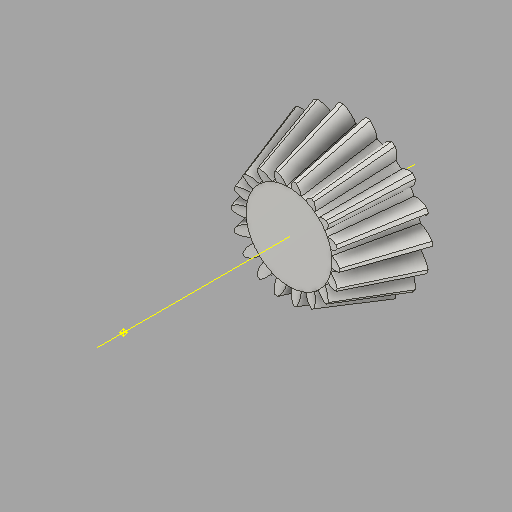
# Autodesk Inventor part: Bevel Gear1
Saved by Autodesk Inventor 2024 (Build 280153000, 153)
## iProperties
Created: 2024-04-12
Part Number: Bevel Gear1
Material: Steel, Mild
Document SubType Name: Modeling
Designer: Alex
Categories: <?xml version="1.0" encoding="UTF-16"?> <MemberInstance><Categories><FamilyTemplate><FamilyTemplateParameter ValueType="xs:double" Id="1" ObjectReferenceKey="da_z" ObjectType="kUserParameterObject"/><FamilyTemplateParameter ValueType="xs:double" Id="2" ObjectReferenceKey="da_b" ObjectType="kUserParameterObject"/><FamilyTemplateParameter ValueType="xs:double" Id="3" ObjectReferenceKey="da_beta" ObjectType="kUserParameterObject"/><FamilyTemplateParameter ValueType="xs:double" Id="4" ObjectReferenceKey="da_dae" ObjectType="kUserParameterObject"/><FamilyTemplateParameter ValueType="xs:double" Id="5" ObjectReferenceKey="da_ve" ObjectType="kUserParameterObject"/><FamilyTemplateParameter ValueType="xs:double" Id="6" ObjectReferenceKey="da_omega" ObjectType="kUserParameterObject"/><FamilyTemplateParameter ValueType="xs:string" Id="7" ObjectReferenceKey="EAIAABAAAAAAHwAAAAAAAIAAAAAAAAAA" ObjectType="83914240" SubObjectId="SurfaceGeometry"/></FamilyTemplate><ParamToTemplateMap><ParamToTemplate CategoryParameter="//CategoryParameter[@InternalName='046C89C9-8512-4d59-83FE-43B91F4F132A']" TemplateParameter="1"/><ParamToTemplate CategoryParameter="//CategoryParameter[@InternalName='2552DF32-E462-4b46-AEBF-C6C7768E72AC']" TemplateParameter="2"/><ParamToTemplate CategoryParameter="//CategoryParameter[@InternalName='C9EE641D-15FC-4fae-A226-E94C4372FDD7']" TemplateParameter="3"/><ParamToTemplate><ParamToTemplate CategoryParameter="//CategoryParameter[@InternalName='00B6519A-459B-49c7-AD84-2E56D39A5744']" ConstantValue="0.000000"/></ParamToTemplate><ParamToTemplate><ParamToTemplate CategoryParameter="//CategoryParameter[@InternalName='04B31F0E-C7A6-4894-AA32-9629BEFACF47']" ConstantValue="1.000000"/></ParamToTemplate><ParamToTemplate><ParamToTemplate CategoryParameter="//CategoryParameter[@InternalName='43CBEC2E-7847-49e7-A936-2F7889FCB2D9']" ConstantValue="0.200000"/></ParamToTemplate><ParamToTemplate><ParamToTemplate CategoryParameter="//CategoryParameter[@InternalName='B1EFC894-105D-4ebd-86BF-FA20ED196853']" ConstantValue="0.300000"/></ParamToTemplate><ParamToTemplate><ParamToTemplate CategoryParameter="//CategoryParameter[@InternalName='51175063-3D10-4879-93E8-6246FE8B403D']" ConstantValue="2060000000.000000"/></ParamToTemplate><ParamToTemplate><ParamToTemplate CategoryParameter="//CategoryParameter[@InternalName='A3A52E27-4454-46a9-B0BD-C932399B70AF']" ConstantValue="0.300000"/></ParamToTemplate><ParamToTemplate CategoryParameter="//CategoryParameter[@InternalName='2A200944-5A8C-41ca-B96E-8520D2E510F1']" TemplateParameter="4"/><ParamToTemplate><ParamToTemplate CategoryParameter="//CategoryParameter[@InternalName='1A637F62-92C8-44bc-B81F-10802510B579']" ConstantValue="2.794076"/></ParamToTemplate><ParamToTemplate CategoryParameter="//CategoryParameter[@InternalName='B52DD4BE-6863-48fb-BF58-89EF6F9EC65C']" TemplateParameter="5"/><ParamToTemplate><ParamToTemplate CategoryParameter="//CategoryParameter[@InternalName='3956BFF2-84D2-457d-93C2-9B0613DEBA67']" ConstantValue="4.168551"/></ParamToTemplate><ParamToTemplate CategoryParameter="//CategoryParameter[@InternalName='739CFA02-461B-4bf8-8049-181FCAD8B28F']" TemplateParameter="6"/><ParamToTemplate><ParamToTemplate CategoryParameter="//CategoryParameter[@InternalName='A27E999F-E2CE-4481-8A2A-EBF499C4C3C5']" ConstantValue="0.000000"/></ParamToTemplate><ParamToTemplate><ParamToTemplate CategoryParameter="//CategoryParameter[@InternalName='9E1B4470-B2D3-4ff1-B813-535BB4CDF51A']" ConstantValue="3520000.000000"/></ParamToTemplate><ParamToTemplate><ParamToTemplate CategoryParameter="//CategoryParameter[@InternalName='F8452263-BFF6-458c-9FB1-07C4B99E95CD']" ConstantValue="11400000.000000"/></ParamToTemplate><ParamToTemplate><ParamToTemplate CategoryParameter="//CategoryParameter[@InternalName='3E3BB259-FD49-497f-8171-6EBC954A3479']" ConstantValue="2.000000"/></ParamToTemplate><ParamToTemplate CategoryParameter="//CategoryParameter[@InternalName='27C3BAF2-7550-4e4b-AE2C-0DB134B7D9B7']" TemplateParameter="7"/></ParamToTemplateMap><Category DisplayName="Gear" InternalName="DC85795E-93AB-48d5-8EEE-5A27447B64BD" Mnemonic="Gear"><CategoryParameter DisplayName="z" InternalName="046C89C9-8512-4d59-83FE-43B91F4F132A" Mnemonic="z"/><CategoryParameter DisplayName="b" InternalName="2552DF32-E462-4b46-AEBF-C6C7768E72AC" Mnemonic="b"/><CategoryParameter DisplayName="||b|" InternalName="C9EE641D-15FC-4fae-A226-E94C4372FDD7" Mnemonic="beta"/><CategoryParameter DisplayName="x" InternalName="00B6519A-459B-49c7-AD84-2E56D39A5744" Mnemonic="x"/><CategoryParameter DisplayName="a*" InternalName="04B31F0E-C7A6-4894-AA32-9629BEFACF47" Mnemonic="a"/><CategoryParameter DisplayName="c*" InternalName="43CBEC2E-7847-49e7-A936-2F7889FCB2D9" Mnemonic="c"/><CategoryParameter DisplayName="r|.f|*" InternalName="B1EFC894-105D-4ebd-86BF-FA20ED196853" Mnemonic="rf"/><CategoryParameter DisplayName="E" InternalName="51175063-3D10-4879-93E8-6246FE8B403D" Mnemonic="E"/><CategoryParameter DisplayName="||m|" InternalName="A3A52E27-4454-46a9-B0BD-C932399B70AF" Mnemonic="mi"/><Category DisplayName="BevelGear" InternalName="0C98F69A-0C2B-4791-B2FE-7691BB227E77" Mnemonic="BevelGear"><CategoryParameter DisplayName="d|.ae|" InternalName="2A200944-5A8C-41ca-B96E-8520D2E510F1" Mnemonic="dae"/><CategoryParameter DisplayName="d|.ai|" InternalName="1A637F62-92C8-44bc-B81F-10802510B579" Mnemonic="dai"/><CategoryParameter DisplayName="A|.e|" InternalName="B52DD4BE-6863-48fb-BF58-89EF6F9EC65C" Mnemonic="ve"/><CategoryParameter DisplayName="A|.i|" InternalName="3956BFF2-84D2-457d-93C2-9B0613DEBA67" Mnemonic="vi"/><CategoryParameter DisplayName="||S|" InternalName="739CFA02-461B-4bf8-8049-181FCAD8B28F" Mnemonic="omega"/><CategoryParameter DisplayName="x|.t|" InternalName="A27E999F-E2CE-4481-8A2A-EBF499C4C3C5" Mnemonic="xt"/><CategoryParameter DisplayName="||s||.Flim|" InternalName="9E1B4470-B2D3-4ff1-B813-535BB4CDF51A" Mnemonic="sFlim"/><CategoryParameter DisplayName="||s||.Hlim|" InternalName="F8452263-BFF6-458c-9FB1-07C4B99E95CD" Mnemonic="sHlim"/><CategoryParameter DisplayName="type" InternalName="3E3BB259-FD49-497f-8171-6EBC954A3479" Mnemonic="type"/><CategoryParameter DisplayName="PitchDiameter" InternalName="27C3BAF2-7550-4e4b-AE2C-0DB134B7D9B7" Mnemonic="IDS_PITCHDIAM"/></Category></Category></Categories></MemberInstance>
Mass: 60.9118 g
Surface Area: 34.3074 cm^2
Volume: 7.7496 cm^3
Density: 7.86 g/cm^3
Appearance: Steel
CustomPartVersion: 1
Author: Alex
Autodesk Inventor part; units mm, degrees
ref_plane "Mesh Plane2" through (0, 0, 0) normal (0.9848078, 0.1736482, 0) x (0, 0, 1)
sketch "Teeth Body Sketch" plane through (0, 0, 0) normal (1, 0, 0) x (0, 1, 0)
  line L0 (0, 0) -> (15.701217, -60.689635) construction
  line L1 (15.701217, -60.689635) -> (19.915653, -59.425304)
  line L2 (19.915653, -59.425304) -> (0, 0) construction
  line L3 (18, -60) -> (0, 0) construction
  line L4 (11.01405, -42.572412) -> (13.970382, -41.685512)
  line L5 (15.701217, -60.689635) -> (11.01405, -42.572412)
  line L6 (19.915653, -59.425304) -> (13.970382, -41.685512)
  line L7 (0, -39.386751) -> (0, 6.564458)
  line L8 (0, -60) -> (19.915653, -60) construction
  dimension "d0" = 36
  dimension "d1" = 31.40243
  dimension "d2" = 39.83131
  dimension "d3" = 18.7
  dimension "d4" = 59.4253
  constraints: 16 end point, 4 point on line, 3 perpendicular, 2 collinear, 1 horizontal alignment, 1 vertical alignment
  measures "d0" diameter of L3.start L7
  measures "d1" diameter of L0.end L7
  measures "d2" diameter of L1.end L7
  measures "d3" distance between parallel lines of L1 L4
  measures "d4" vertical distance of L1.end L0.start
revolve "Teeth Body" add sketch "Teeth Body Sketch" angle 360 about axis through (0, 0, 0) along (0, 0, 1)
ref_plane "Tooth Plane" through (0, 18, -60) normal (0, -0.2873479, 0.9578263) x (1, 0, 0)
sketch "Start Sketch" plane through (0, 18, -60) normal (0, -0.2873479, 0.9578263) x (1, 0, 0)
  line L0 (0, -23.505131) -> (0, 10.644758)
  arc A0 (-0.8854, -2.928) -> (-4.272774, 2.903262) centre (-7.980511, -3.15005) ccw
  arc A1 (4.272774, 2.903262) -> (0.8854, -2.928) centre (7.980511, -3.15005) ccw
  line L1 (-0.8854, -2.928) -> (0.8854, -2.928)
  arc A2 (4.272774, 2.903262) -> (-4.272774, 2.903262) centre (0, -18.792552) ccw
  dimension "d7" = 7.09858
  dimension "d8" = 7.98051
  dimension "d9" = 15.6425
  dimension "d57" = 22.11255
  dimension "d58" = 15.86455
  constraints: 6 point on circle, 3 centre point, 3 symmetric about line, 2 end point, 1 coincident, 1 perpendicular, 1 other
  measures "d7" radius of A0
  measures "d8" horizontal distance of point (0, -18.793) A0.centre
  measures "d9" vertical distance of point (0, -18.793) A0.centre
  measures "d57" radius of A2
  measures "d58" distance from line of A2.centre L1
sketch "End Sketch" plane through (0, 12.563378, -41.877927) normal (0, -0.2873479, 0.9578263) x (1, 0, 0)
  line L0 (0, -15.35404) -> (0, 6.953444)
  arc A0 (-0.617979, -2.043643) -> (-2.982248, 2.026377) centre (-5.570121, -2.198626) ccw
  arc A1 (2.982248, 2.026377) -> (0.617979, -2.043643) centre (5.570121, -2.198626) ccw
  line L1 (-0.617979, -2.043643) -> (0.617979, -2.043643)
  arc A2 (2.982248, 2.026377) -> (-2.982248, 2.026377) centre (0, -13.116552) ccw
  dimension "d12" = 4.95457
  dimension "d15" = 5.57012
  dimension "d16" = 10.91793
  dimension "d59" = 15.4338
  dimension "d60" = 11.07291
  constraints: 6 point on circle, 3 centre point, 3 symmetric about line, 2 end point, 1 coincident, 1 other
  measures "d12" radius of A0
  measures "d15" horizontal distance of A0.centre point (0, -13.117)
  measures "d16" vertical distance of A0.centre point (0, -13.117)
  measures "d59" radius of A2
  measures "d60" distance from line of A2.centre L1
loft "Loft" cut profiles "Start Sketch", "End Sketch"
pattern_circular "Circular Pattern" count 18 over 360 about axis through (0, 0, 0) along (0, 0, 1) of "Loft"
ref_plane "End Plane" through (0, 12.563378, -41.877927) normal (0, -0.2873479, 0.9578263) x (1, 0, 0)
sketch3d "3D Sketch Right"
ref_plane "End Plane Right" through (-5.461188, 11.314322, -41.877927) normal (0.1249076, -0.2587797, 0.9578263) x (0.9005796, 0.4346911, 0)
sketch "End Sketch Right" plane through (-5.461188, 11.314322, -41.877927) normal (0.1249076, -0.2587797, 0.9578263) x (0.9005796, 0.4346911, 0)
  arc A0 (-0.617979, -2.043643) -> (-2.982248, 2.026377) centre (-5.570121, -2.198626) ccw
  line L0 (0, -23.41048) -> (0, 14.060583)
  arc A1 (2.982248, 2.026377) -> (0.617979, -2.043643) centre (5.570121, -2.198626) ccw
  line L1 (-0.617979, -2.043643) -> (0.617979, -2.043643)
  arc A2 (2.982248, 2.026377) -> (-2.982248, 2.026377) centre (0, -13.116552) ccw
  dimension "d70" = 5.57012
  dimension "d71" = 10.91793
  dimension "d72" = 4.95457
  dimension "d73" = 11.07291
  dimension "d74" = 15.4338
  constraints: 6 point on circle, 3 centre point, 3 symmetric about line, 2 end point, 1 coincident, 1 perpendicular, 1 other
  measures "d70" horizontal distance of A2.centre A0.centre
  measures "d71" vertical distance of point (0, -13.117) A0.centre
  measures "d72" radius of A0
  measures "d73" distance from line of point (0, -13.117) L1
  measures "d74" radius of A2
feature "Loft Right" [suppressed]
pattern_circular "Circular Pattern Right" [suppressed]
sketch3d "3D Sketch Left"
ref_plane "End Plane Left" through (5.430211, 11.314322, -41.86862) normal (-0.1242353, -0.2588553, 0.9578933) x (0.9015437, -0.4326881, 0)
sketch "End Sketch Left" plane through (5.430211, 11.314322, -41.86862) normal (-0.1242353, -0.2588553, 0.9578933) x (0.9015437, -0.4326881, 0)
  line L0 (0, -39.461099) -> (0, 22.438376)
  arc A0 (-0.617979, -2.033445) -> (-2.982248, 2.036574) centre (-5.570121, -2.188428) ccw
  arc A1 (2.982248, 2.036574) -> (0.617979, -2.033445) centre (5.570121, -2.188428) ccw
  line L1 (-0.617979, -2.033445) -> (0.617979, -2.033445)
  ellipse E0 centre (0, -11.968931) end of major axis (13.970382, -11.968931) minor radius 13.382135
  arc A2 (2.982248, 2.036574) -> (-2.982248, 2.036574) centre (0, -13.106354) ccw
  dimension "d56" = 13.38213
  dimension "d30" = 4.95457
  dimension "d31" = 5.57012
  dimension "d32" = 10.91793
  dimension "d61" = 15.4338
  dimension "d62" = 11.07291
  constraints: 6 point on circle, 3 centre point, 3 symmetric about line, 2 end point, 1 coincident, 2 other
  measures "d30" radius of A0
  measures "d31" horizontal distance of point (0, -13.106) A0.centre
  measures "d32" vertical distance of A0.centre point (0, -13.106)
  measures "d61" radius of A2
  measures "d62" distance from line of point (0, -13.106) L1
feature "Loft Left" [suppressed]
pattern_circular "Circular Pattern Left" [suppressed]
sketch "Body Sketch" plane through (0, 0, 0) normal (1, 0, 0) x (0, 1, 0)
  line L0 (0, -35.037536) -> (0, -19.530831)
  line L1 (15.701217, -60.689635) -> (11.01405, -42.572412)
  line L2 (11.01405, -42.572412) -> (0, -42.572412)
  line L3 (15.701217, -60.689635) -> (0, -60.689635)
  constraints: 4 end point, 2 perpendicular, 2 point on line
sketch "Body Sketch outline for Fix Body" plane through (0, 0, 0) normal (1, 0, 0) x (0, 1, 0)
  line L0 (0, -60.689635) -> (15.701217, -60.689635)
  line L1 (0, -42.572412) -> (0, -60.689635)
  line L2 (11.01405, -42.572412) -> (0, -42.572412)
  line L3 (15.701217, -60.689635) -> (11.01405, -42.572412)
revolve "Fix Body" add sketch "Body Sketch outline for Fix Body" angle 360 about axis through (0, 0, 0) along (0, 0, 1)
sketch "Sketch6" plane through (0, 0, 0) normal (1, 0, 0) x (0, 1, 0)
  line L0 (18, -60) -> (0, 0)
  line L1 (0, -37.799919) -> (0, 6.299986)
surface revolve "Pitch Diameter" sketch "Sketch6" angle 360 about axis through (0, 0, 0) along (0, 0, 1) shown no curves L0
equation "\"d0\" = da_de"
equation "\"d1\" = da_dfe"
equation "\"d2\" = da_dae"
equation "\"d3\" = da_b"
equation "\"d4\" = da_ve"
equation "\"d7\" = fd_rr"
equation "\"d8\" = fd_x"
equation "\"d9\" = fd_y"
equation "\"d57\" = 0.5 * fd_dva + 0.3 * da_he"
equation "\"d58\" = 0.5 * fd_dva - 1.12 * da_he"
equation "\"da_teethtype\" = 0"
equation "\"da_b\" = 18.7"
equation "\"da_de\" = 36"
equation "\"da_dae\" = 39.83131"
equation "\"da_dfe\" = 31.40243"
equation "\"da_le\" = 62.64184"
equation "\"da_omega\" = 90deg"
equation "\"da_beta\" = 0"
equation "\"da_delta\" = 16.699244deg"
equation "\"da_alpha\" = 20deg"
equation "\"da_he\" = 4.4"
equation "\"da_ve\" = 59.4253"
equation "\"da_zv\" = 18.792552"
equation "\"fd_loft\" = da_b + 0.05 * da_he"
equation "\"fd_x\" = fd_x1 + fd_x2"
equation "\"fd_y\" = fd_y1 - fd_y2"
equation "\"fd_dd\" = fd_dva - 0.8 * da_he"
equation "\"da_dvw\" = 37.5851"
equation "\"d11\" = fd_loft"
equation "\"da_dm\" = 30.62659"
equation "\"da_x\" = 0"
equation "\"da_m\" = 2"
equation "\"d50\" = da_omega"
equation "\"fd_rr\" = 7.098584"
equation "\"fd_dva\" = 41.585103"
equation "\"fd_x1\" = 1.58636"
equation "\"fd_x2\" = 6.394151"
equation "\"fd_y1\" = 18.725476"
equation "\"fd_y2\" = 3.082974"
body "Solid1"
body "Srf1"
